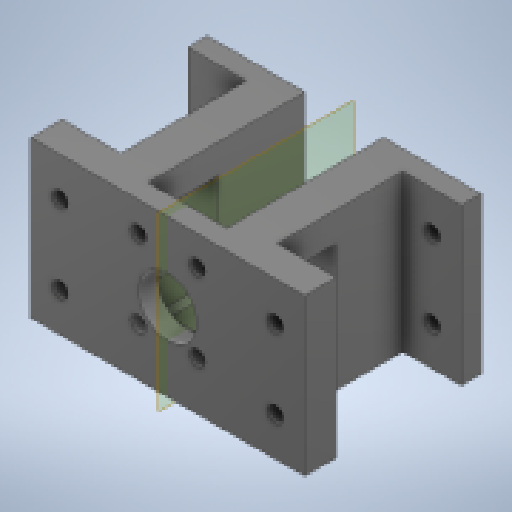
# Autodesk Inventor part: motor1_bracket
Saved by Autodesk Inventor 2026.2 (Build 302298010, 298A)
## iProperties
Created: 2026-04-11
Part Number: motor1_bracket
Material: ABS Plastic
Document SubType Name: Modeling
Designer: chris
Density: 1.06 g/cm^3
Appearance: Smooth - White
Author: chris
Autodesk Inventor part; units mm, degrees
ref_plane "YZ Plane" through (0, 0, 0) normal (1, 0, 0) x (0, 1, 0)
ref_plane "XZ Plane" through (0, 0, 0) normal (0, 1, 0) x (-1, 0, 0)
ref_plane "XY Plane" through (0, 0, 0) normal (0, 0, 1) x (1, 0, 0)
sketch "Sketch1" plane through (0, 0, 0) normal (0, 0, 1) x (1, 0, 0)
  line L0 (-20, -20) -> (20, -20)
  line L1 (20, -20) -> (20, 20)
  line L2 (20, 20) -> (-20, 20)
  line L3 (-20, 20) -> (-20, -20)
  line L4 (-20, -20) -> (20, 20) construction
  line L5 (20, -20) -> (-20, 20) construction
  point P0 (0, 0)
  dimension "d0" = 40
  dimension "d1" = 40
  constraints: 12 end point, 2 midpoint, 2 parallel, 1 horizontal, 1 perpendicular
  measures "d0" distance of L2.end L1.end
  measures "d1" distance of L1.end L0.end
extrude "Extrusion1" add sketch "Sketch1" along normal blind 5
sketch "Sketch3" plane through (0, 0, 0) normal (0, 0, -1) x (-1, 0, 0)
  line L0 (-20, -20) -> (20, -20)
  line L1 (20, -20) -> (20, 20)
  line L2 (20, 20) -> (-20, 20)
  line L3 (-20, 20) -> (-20, -20)
  line L4 (-20, -20) -> (20, 20) construction
  line L5 (20, -20) -> (-20, 20) construction
  line L6 (-10.1, -10) -> (10.1, -10)
  line L7 (10.1, -10) -> (10.1, 20)
  line L8 (10.1, 20) -> (-10.1, 20)
  line L9 (-10.1, 20) -> (-10.1, -10)
  line L10 (-10.1, -10) -> (10.1, 20) construction
  line L11 (10.1, -10) -> (-10.1, 20) construction
  point P0 (0, 0)
  point P1 (0, 5)
  dimension "d8" = 40
  dimension "d9" = 40
  dimension "d10" = 20.2
  dimension "d11" = 30
  dimension "d55" = 20
  constraints: 24 end point, 4 midpoint, 4 parallel, 2 horizontal, 2 perpendicular, 1 point on line
  measures "d8" distance of L2.end L1.end
  measures "d9" distance of L1.end L0.end
  measures "d10" distance of L6.start L6.end
  measures "d11" distance of L6.end L7.end
  measures "d55" distance from line of L1 point (0, 5)
extrude "Extrusion3" add sketch "Sketch3" along normal blind 40.1 contours L3 L2 L9 L6 L7 L1 L0
sketch "Sketch4" plane through (0, 0, 0) normal (0, 0, -1) x (-1, 0, 0)
  circle A0 centre (0, 0) radius 7.5
  dimension "d14" = 15
  constraints: 1 centre point, 1 coincident
  measures "d14" diameter of A0
extrude "Extrusion4" cut sketch "Sketch4" against normal blind 6
sketch "Sketch6" plane through (20, -20, -40.1) normal (1, 0, 0) x (0, 0, -1)
  line L0 (-45.1, 40) -> (-37.1, 40)
  line L1 (-37.1, 40) -> (-37.1, 0)
  line L2 (-37.1, 0) -> (-45.1, 0)
  line L3 (-45.1, 0) -> (-45.1, 40)
  line L4 (-45.1, 40) -> (-37.1, 0) construction
  line L5 (-37.1, 40) -> (-45.1, 0) construction
  line L6 (0, 40) -> (-45.1, 40) projected
  line L7 (-45.1, 0) -> (0, 0) projected
  line L8 (-45.1, 0) -> (-45.1, 40) projected
  point P0 (-40.1, 20)
  point P1 (-41.1, 20)
  point P2 (-40.1, 40)
  point P3 (-45.1, 50)
  dimension "d19" = 8
  constraints: 12 end point, 3 collinear, 2 midpoint, 2 parallel, 1 horizontal, 1 perpendicular
  measures "d19" distance of L1.end L2.end
extrude "Extrusion6" add sketch "Sketch6" along normal blind 15
mirror "Mirror1" about plane through (0, 0, 0) normal (1, 0, 0) of "Extrusion6"
sketch "Sketch7" plane through (0, 0, 5) normal (0, 0, 1) x (1, 0, 0)
  circle A0 centre (27.5, 10) radius 2.05
  circle A1 centre (27.5, -10) radius 2.05
  circle A2 centre (-27.5, -10) radius 2.05
  circle A3 centre (-27.5, 10) radius 2.05
  line L0 (35, 20) -> (35, -20) projected
  line L1 (-35, 20) -> (-35, -20) projected
  line L2 (35, -20) -> (-35, -20) projected
  line L3 (-35, 20) -> (35, 20) projected
  line L4 (-20, 20) -> (-35, 20) projected
  point P0 (0, 0)
  point P1 (20, 20)
  dimension "d22" = 4.1
  dimension "d23" = 4.1
  dimension "d24" = 4.1
  dimension "d25" = 4.1
  dimension "d26" = 7.5
  dimension "d27" = 7.5
  dimension "d28" = 7.5
  dimension "d29" = 7.5
  dimension "d30" = 10
  dimension "d31" = 10
  dimension "d32" = 10
  dimension "d33" = 10
  constraints: 4 centre point
  measures "d22" diameter of A0
  measures "d23" diameter of A1
  measures "d24" diameter of A2
  measures "d25" diameter of A3
  measures "d26" distance from line of L0 A0.centre
  measures "d27" distance from line of L0 A1.centre
  measures "d28" distance from line of L1 A3.centre
  measures "d29" distance from line of L1 A2.centre
  measures "d30" distance from line of L2 A2.centre
  measures "d31" distance from line of L2 A1.centre
  measures "d32" distance from line of L3 A0.centre
  measures "d33" distance from line of L4 A3.centre
extrude "Extrusion7" cut sketch "Sketch7" against normal blind 45.1 contours A0 | A1 | A2 | A3
sketch "Sketch9" plane through (20, -20, -3) normal (0, 0, -1) x (-1, 0, 0)
  circle A0 centre (-7.5, 30) radius 2.05 projected
  circle A1 centre (-7.5, 10) radius 2.05 projected
  circle A2 centre (47.5, 30) radius 2.05 projected
  circle A3 centre (47.5, 10) radius 2.05 projected
  circle A4 centre (-7.5, 30) radius 5
  circle A5 centre (-7.5, 10) radius 5
  circle A6 centre (47.5, 30) radius 5
  circle A7 centre (47.5, 10) radius 5
  point P0 (20, 20)
  dimension "d39" = 10
  dimension "d40" = 10
  dimension "d41" = 10
  dimension "d42" = 10
  constraints: 4 centre point, 4 coincident
  measures "d39" diameter of A4
  measures "d40" diameter of A5
  measures "d41" diameter of A6
  measures "d42" diameter of A7
extrude "Extrusion8" cut sketch "Sketch9" against normal blind 5 contours A0 | A1 | A4 | A5 | A6 | A7
sketch "Sketch10" plane through (-20, -20, -40.1) normal (-1, 0, 0) x (0, 0, 1)
  line L0 (22.1, 17.5) -> (37.1, 17.5)
  line L1 (37.1, 17.5) -> (37.1, 32.5)
  line L2 (37.1, 32.5) -> (22.1, 32.5)
  line L3 (22.1, 32.5) -> (22.1, 17.5)
  line L4 (22.1, 17.5) -> (37.1, 32.5) construction
  line L5 (37.1, 17.5) -> (22.1, 32.5) construction
  line L6 (37.1, 0) -> (37.1, 40) projected
  line L7 (40.1, 10) -> (0, 10) projected
  point P0 (40.1, 20)
  point P1 (29.6, 25)
  dimension "d45" = 15
  dimension "d46" = 15
  dimension "d47" = 7.5
  constraints: 12 end point, 2 midpoint, 2 parallel, 1 collinear, 1 horizontal, 1 perpendicular
  measures "d45" distance of L2.end L1.end
  measures "d46" distance of L1.end L0.end
  measures "d47" distance between parallel lines of L7 L0
extrude "Extrusion9" cut sketch "Sketch10" against normal through all
sketch "Sketch11" plane through (-20, -20, -40.1) normal (0, -1, 0) x (1, 0, 0)
  line L0 (27.5, 22.1) -> (12.5, 22.1)
  line L1 (12.5, 22.1) -> (12.5, 37.1)
  line L2 (12.5, 37.1) -> (27.5, 37.1)
  line L3 (27.5, 37.1) -> (27.5, 22.1)
  line L4 (27.5, 22.1) -> (12.5, 37.1) construction
  line L5 (12.5, 22.1) -> (27.5, 37.1) construction
  line L6 (0, 37.1) -> (-15, 37.1) projected
  line L7 (0, 0) -> (0, 37.1) projected
  point P0 (20, 40.1)
  point P1 (20, 29.6)
  dimension "d50" = 15
  dimension "d51" = 15
  dimension "d52" = 20
  constraints: 12 end point, 2 midpoint, 2 parallel, 1 collinear, 1 horizontal, 1 perpendicular
  measures "d50" distance of L1.end L2.end
  measures "d51" distance of L0.end L1.end
  measures "d52" distance from line of L7 point (20, 29.6)
extrude "Extrusion10" cut sketch "Sketch11" against normal through all
sketch "Sketch12" plane through (0, 0, 0) normal (0, 0, -1) x (-1, 0, 0)
  ellipse E0 centre (7.952, -7.882) end of major axis (8.818, -8.748) minor radius 1 (8.1756, -9) -> (9.07, -8.1056) ccw projected
  line L0 (-8.1756, -9) -> (8.1756, -9) projected
  ellipse E1 centre (-7.952, -7.882) end of major axis (-8.818, -8.748) minor radius 1 (-9.07, -8.1056) -> (-8.1756, -9) ccw projected
  line L1 (-9.07, 28.2056) -> (-9.07, -8.1056) projected
  ellipse E2 centre (-7.952, 27.982) end of major axis (-8.818, 28.848) minor radius 1 (-8.1756, 29.1) -> (-9.07, 28.2056) ccw projected
  line L2 (8.1756, 29.1) -> (-8.1756, 29.1) projected
  ellipse E3 centre (7.952, 27.982) end of major axis (8.818, 28.848) minor radius 1 (9.07, 28.2056) -> (8.1756, 29.1) ccw projected
  line L3 (9.07, -8.1056) -> (9.07, 28.2056) projected
  circle A0 centre (-7.525, 27.6) radius 0.7835 projected
  circle A1 centre (7.525, 27.6) radius 0.7835 projected
  circle A2 centre (-7.525, 12.5) radius 0.7835 projected
  circle A3 centre (7.525, 12.5) radius 0.7835 projected
  circle A4 centre (-7.525, -7.5) radius 0.7835 projected
  circle A5 centre (7.525, -7.5) radius 0.7835 projected
  circle A6 centre (0, 0) radius 6.4 projected
  point P0 (0, 0)
  constraints: 4 other
hole "Hole1" at (-7.525, -7.5, 0) at (-7.525, 12.5, 0) at (7.525, 12.5, 0) at (7.525, -7.5, 0) direction (0, 0, 1) diameter 2.1 end through all
sketch "Sketch13" plane through (0, 0, 5) normal (0, 0, 1) x (1, 0, 0)
  circle A0 centre (-7.525, 12.5) radius 1.05 projected
  circle A1 centre (7.525, 12.5) radius 1.05 projected
  circle A2 centre (-7.525, 12.5) radius 2
  circle A3 centre (7.525, 12.5) radius 2
  point P0 (0, 0)
  dimension "d63" = 4
  dimension "d64" = 4
  constraints: 2 centre point, 2 coincident
  measures "d63" diameter of A2
  measures "d64" diameter of A3
extrude "Extrusion11" cut sketch "Sketch13" against normal blind 2.5 contours A0 | A1 | A2 | A3
mirror "Mirror2" about plane through (0, 0, 0) normal (1, 0, 0)
sketch "Sketch16" plane through (0, 0, -40.1) normal (0, 0, -1) x (-1, 0, 0)
  circle A0 centre (37.5, 12.5) radius 2.05
  line L0 (45, -20) -> (45, 20) projected
  line L1 (10.1, 20) -> (45, 20) projected
  circle A1 centre (37.5, -12.5) radius 2.05
  circle A2 centre (-37.5, 12.5) radius 2.05
  circle A3 centre (-37.5, -12.5) radius 2.05
  line L2 (45, -20) -> (-45, -20) projected
  line L3 (-45, -20) -> (-45, 20) projected
  line L4 (-10.1, 20) -> (-20, 20) projected
  point P0 (0, 0)
  dimension "d74" = 4.1
  dimension "d75" = 7.5
  dimension "d76" = 7.5
  dimension "d77" = 4.1
  dimension "d78" = 4.1
  dimension "d79" = 4.1
  dimension "d80" = 7.5
  dimension "d81" = 7.5
  dimension "d82" = 7.5
  dimension "d83" = 7.5
  dimension "d84" = 7.5
  dimension "d85" = 7.5
  constraints: 4 centre point
  measures "d74" diameter of A0
  measures "d75" distance from line of L0 A0.centre
  measures "d76" distance from line of L1 A0.centre
  measures "d77" diameter of A1
  measures "d78" diameter of A2
  measures "d79" diameter of A3
  measures "d80" distance from line of L0 A1.centre
  measures "d81" distance from line of L2 A1.centre
  measures "d82" distance from line of L3 A3.centre
  measures "d83" distance from line of L2 A3.centre
  measures "d84" distance from line of L4 A2.centre
  measures "d85" distance from line of L3 A2.centre
extrude "Extrusion14" cut sketch "Sketch16" against normal through all
sketch "Sketch18" plane through (0, 0, 5) normal (0, 0, 1) x (1, 0, 0)
  circle A0 centre (7.525, -7.5) radius 1.05 projected
  circle A1 centre (-7.525, -7.5) radius 1.05 projected
  circle A2 centre (7.525, -7.5) radius 2
  circle A3 centre (-7.525, -7.5) radius 2
  point P0 (0, 0)
  dimension "d94" = 4
  dimension "d95" = 4
  constraints: 2 centre point, 2 coincident
  measures "d94" diameter of A2
  measures "d95" diameter of A3
extrude "Extrusion16" cut sketch "Sketch18" against normal blind 2.5
sketch "Sketch19" plane through (0, 0, -40.1) normal (0, 0, -1) x (-1, 0, 0)
  line L0 (20, 20) -> (20, -20)
  line L1 (20, -20) -> (35, -20)
  line L2 (35, -20) -> (35, 20)
  line L3 (-35, -20) -> (-20, -20)
  line L4 (-20, -20) -> (-20, 20)
  line L5 (-20, 20) -> (-35, 20)
  line L6 (-35, 20) -> (-35, -20)
  line L7 (-35, -20) -> (-20, 20) construction
  line L8 (-20, -20) -> (-35, 20) construction
  line L9 (20, 20) -> (35, 20)
  line L10 (20, -20) -> (20, 20) projected
  line L11 (20, 20) -> (35, 20) projected
  line L12 (35, -20) -> (35, 20) projected
  line L13 (20, -20) -> (35, -20) projected
  line L14 (-20, 20) -> (-20, -20) projected
  line L15 (-20, 20) -> (-35, 20) projected
  line L16 (-35, -20) -> (-35, 20) projected
  line L17 (-20, -20) -> (-35, -20) projected
  point P0 (0, 0)
  point P1 (-27.5, 0)
  constraints: 20 end point, 8 collinear, 3 perpendicular, 2 horizontal, 2 midpoint, 2 parallel, 1 vertical
extrude "Extrusion17" add sketch "Sketch19" against normal blind 5
sketch "Sketch20" plane through (0, 0, -40.1) normal (0, 0, -1) x (-1, 0, 0)
  circle A0 centre (-27.5, 10) radius 2.05 projected
  circle A1 centre (-27.5, -10) radius 2.05 projected
  circle A2 centre (27.5, -10) radius 2.05 projected
  circle A3 centre (27.5, 10) radius 2.05 projected
  circle A4 centre (-27.5, 10) radius 2.05
  circle A5 centre (-27.5, -10) radius 2.05
  circle A6 centre (27.5, 10) radius 2.05
  circle A7 centre (27.5, -10) radius 2.05
  point P0 (0, 0)
  constraints: 4 centre point, 4 coincident, 4 concentric
extrude "Extrusion18" cut sketch "Sketch20" against normal blind 10
ref_plane "Work Plane1" through (0, 0, 0) normal (1, 0, 0) x (0, 1, 0)
body "Solid1"
